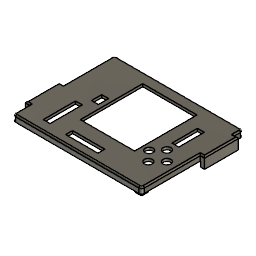
_Top Cover HiLetGo LCD.2d9b06c0-f316-4b58-bc27-3410c5de609b (Autodesk Fusion 360 design; units mm, degrees)
Autodesk Fusion 360 part; units mm, degrees
imported_body "Derived Base Feature2" makes body 1
imported_body "Derived Base Feature3" makes body 2
imported_body "Derived Base Feature4" makes body 3
imported_body "Derived Base Feature5" makes body 4
imported_body "Derived Base Feature6" makes body 5
imported_body "Derived Base Feature7" makes body 6
imported_body "Source Assembly: Context1(Enclosure)" makes body 7
sketch "Sketch1" plane through (0, 0, 38.1) normal (0, 0, 1) x (-1, 0, 0)
  line L0 (59.055, -28.1321) -> (60.325, -26.8621)
  line L1 (60.325, -26.8621) -> (60.325, -7.8121)
  line L2 (60.325, -7.8121) -> (59.055, -6.5421)
  line L3 (59.055, -6.5421) -> (59.055, 11.6667)
  arc A0 (59.055, 11.6667) -> (57.785, 12.9367) centre (57.785, 11.6667) ccw
  line L4 (57.785, 12.9367) -> (-57.785, 12.9367)
  arc A1 (-57.785, 12.9367) -> (-59.055, 11.6667) centre (-57.785, 11.6667) ccw
  line L5 (-59.055, 11.6667) -> (-59.055, -42.6733)
  line L6 (-59.055, -42.6733) -> (-60.325, -43.9433)
  line L7 (-60.325, -43.9433) -> (-60.325, -69.3433)
  line L8 (-60.325, -69.3433) -> (-59.055, -70.6133)
  line L9 (-59.055, -70.6133) -> (-59.055, -78.5033)
  arc A2 (-59.055, -78.5033) -> (-57.785, -79.7733) centre (-57.785, -78.5033) ccw
  line L10 (-57.785, -79.7733) -> (57.785, -79.7733)
  arc A3 (57.785, -79.7733) -> (59.055, -78.5033) centre (57.785, -78.5033) ccw
  line L11 (59.055, -78.5033) -> (59.055, -28.1321)
  line L12 (58.15, 12.0317) -> (58.15, -78.8683)
  line L13 (58.15, -78.8683) -> (-58.15, -78.8683)
  line L14 (-58.15, -78.8683) -> (-58.15, 12.0317)
  line L15 (-58.15, 12.0317) -> (58.15, 12.0317)
  line L16 (-57.785, -81.0433) -> (57.785, -81.0433)
  arc A4 (57.785, -81.0433) -> (60.325, -78.5033) centre (57.785, -78.5033) ccw
  line L17 (60.325, -78.5033) -> (60.325, -26.8621)
  line L18 (60.325, -7.8121) -> (60.325, 11.6667)
  arc A5 (60.325, 11.6667) -> (57.785, 14.2067) centre (57.785, 11.6667) ccw
  line L19 (57.785, 14.2067) -> (-57.785, 14.2067)
  arc A6 (-57.785, 14.2067) -> (-60.325, 11.6667) centre (-57.785, 11.6667) ccw
  line L20 (-60.325, 11.6667) -> (-60.325, -43.9433)
  line L21 (-60.325, -69.3433) -> (-60.325, -78.5033)
  arc A7 (-60.325, -78.5033) -> (-57.785, -81.0433) centre (-57.785, -78.5033) ccw
  line L22 (-60.325, -40.7683) -> (-64.2937, -40.7683)
  line L23 (-64.2937, -40.7683) -> (-64.2937, -72.5183)
  line L24 (-64.2937, -72.5183) -> (-60.325, -72.5183)
  line L25 (-60.325, -72.5183) -> (-60.325, -40.7683)
  line L26 (-62.7062, -46.3246) -> (-62.7062, -66.9621)
  line L27 (60.325, -33.2121) -> (64.2937, -33.2121)
  line L28 (64.2937, -33.2121) -> (64.2937, -1.4621)
  line L29 (64.2937, -1.4621) -> (60.325, -1.4621)
  line L30 (60.325, -1.4621) -> (60.325, -33.2121)
  line L31 (62.7063, -24.4808) -> (62.7063, -10.1933)
  line L32 (60.625, -33.2121) -> (60.625, -1.4621)
  line L33 (60.325, -78.8683) -> (60.325, 12.0317)
  line L34 (-60.625, -72.5183) -> (-60.625, -40.7683)
  line L35 (15.0813, -72.1533) -> (-21.4312, -72.1533) construction
  line L36 (-21.4312, -72.1533) -> (-21.4312, -15.0033) construction
  line L37 (-21.4312, -15.0033) -> (15.0813, -15.0033) construction
  line L38 (15.0813, -15.0033) -> (15.0813, -72.1533) construction
  line L39 (15.0813, -65.8033) -> (-21.4312, -65.8033) construction
  line L40 (-21.4312, -65.8033) -> (-21.4312, -26.1158) construction
  line L41 (-21.4312, -26.1158) -> (15.0813, -26.1158) construction
  line L42 (15.0813, -26.1158) -> (15.0813, -65.8033) construction
  line L43 (18.6531, -0.0808) -> (-11.5094, -0.0808)
  line L44 (-11.5094, -0.0808) -> (-11.5094, 6.2692)
  line L45 (-11.5094, 6.2692) -> (18.6531, 6.2692)
  line L46 (18.6531, 6.2692) -> (18.6531, -0.0808)
  line L47 (34.1312, -42.9433) -> (27.7812, -42.9433)
  line L48 (27.7812, -42.9433) -> (27.7812, -33.4183)
  line L49 (27.7812, -33.4183) -> (34.1312, -33.4183)
  line L50 (34.1312, -33.4183) -> (34.1312, -42.9433)
  line L51 (-38.1, -60.4058) -> (-44.45, -60.4058)
  line L52 (-44.45, -60.4058) -> (-44.45, -36.5933)
  line L53 (-44.45, -36.5933) -> (-38.1, -36.5933)
  line L54 (-38.1, -36.5933) -> (-38.1, -60.4058)
  circle A8 centre (-33.3375, -19.9246) radius 3.175
  circle A9 centre (-33.3375, -19.9246) radius 5.5562
  circle A10 centre (-41.275, -28.6558) radius 3.175
  circle A11 centre (-41.275, -28.6558) radius 5.5562
  circle A12 centre (-50.8, -19.1308) radius 3.175
  circle A13 centre (-50.8, -19.1308) radius 5.5562
  circle A14 centre (-42.0687, -10.3996) radius 3.175
  circle A15 centre (-42.0687, -10.3996) radius 5.5562
  circle A16 centre (-41.275, -28.6558) radius 3.675
  circle A17 centre (-33.3375, -19.9246) radius 3.675
  circle A18 centre (-50.8, -19.1308) radius 3.675
  circle A19 centre (-42.0687, -10.3996) radius 3.675
  line L55 (41.275, 4.6817) -> (34.925, 4.6817)
  line L56 (34.925, 4.6817) -> (34.925, -25.4808)
  line L57 (34.925, -25.4808) -> (41.275, -25.4808)
  line L58 (41.275, -25.4808) -> (41.275, 4.6817)
  line L59 (-21.9312, -72.6533) -> (-21.9312, -14.5033) construction
  line L60 (-21.9312, -14.5033) -> (15.5813, -14.5033) construction
  line L61 (15.5813, -14.5033) -> (15.5813, -72.6533) construction
  line L62 (15.5813, -72.6533) -> (-21.9312, -72.6533) construction
  line L63 (57.95, -78.6683) -> (51.6, -78.6683)
  line L64 (51.6, -78.6683) -> (51.6, -76.1283)
  line L65 (51.6, -76.1283) -> (55.41, -76.1283)
  line L66 (57.95, -78.6683) -> (57.95, -72.3183)
  line L67 (57.95, -72.3183) -> (55.41, -72.3183)
  line L68 (55.41, -72.3183) -> (55.41, -76.1283)
  line L69 (51.6, -78.6683) -> (51.6, -78.8683)
  line L70 (57.95, -72.3183) -> (58.15, -72.3183)
  line L71 (85.0596, -33.4183) -> (-85.0118, -33.4183) construction
  line L72 (51.6, 11.8317) -> (51.6, 12.0317)
  line L73 (57.95, 11.8317) -> (51.6, 11.8317)
  line L74 (57.95, 5.4817) -> (55.41, 5.4817)
  line L75 (55.41, 5.4817) -> (55.41, 9.2917)
  line L76 (57.95, 11.8317) -> (57.95, 5.4817)
  line L77 (57.95, 5.4817) -> (58.15, 5.4817)
  line L78 (51.6, 9.2917) -> (55.41, 9.2917)
  line L79 (51.6, 11.8317) -> (51.6, 9.2917)
  line L80 (0, -87.3252) -> (0, 24.4348) construction
  line L81 (-57.95, 5.4817) -> (-58.15, 5.4817)
  line L82 (-57.95, 5.4817) -> (-55.41, 5.4817)
  line L83 (-57.95, 11.8317) -> (-57.95, 5.4817)
  line L84 (-55.41, 5.4817) -> (-55.41, 9.2917)
  line L85 (-51.6, 9.2917) -> (-55.41, 9.2917)
  line L86 (-51.6, 11.8317) -> (-51.6, 9.2917)
  line L87 (-57.95, 11.8317) -> (-51.6, 11.8317)
  line L88 (-51.6, 11.8317) -> (-51.6, 12.0317)
  line L89 (23.8363, -71.0658) -> (-26.9637, -71.0658)
  line L90 (-26.9637, -71.0658) -> (-26.9637, -12.6458)
  line L91 (-26.9637, -12.6458) -> (23.8363, -12.6458)
  line L92 (23.8363, -12.6458) -> (23.8363, -71.0658)
  point P0 (-64.2937, -56.6433)
  point P1 (-62.7062, -56.6433)
  point P2 (64.2937, -17.3371)
  point P3 (62.7063, -17.3371)
  point P4 (58.15, -33.4183)
  point P5 (-58.15, -33.4183)
  point P6 (0, -78.8683)
  dimension "d3" = 31.75
  dimension "d4" = 3.9688
  dimension "d5" = 31.75
  dimension "d6" = 3.9688
  dimension "d9" = 0.3
  dimension "d10" = 0.3
  dimension "d23" = 57.15
  dimension "d24" = 36.5125
  dimension "d25" = 29.21
  dimension "d26" = 38.8938
  dimension "d27" = 39.6875
  dimension "d28" = 11.1125
  dimension "d29" = 6.35
  dimension "d30" = 7.9375
  dimension "d31" = 41.6719
  dimension "d32" = 30.1625
  dimension "d33" = 9.525
  dimension "d34" = 6.35
  dimension "d35" = 47.625
  dimension "d36" = 26.1938
  dimension "d37" = 6.35
  dimension "d38" = 15.875
  dimension "d39" = 23.8125
  dimension "d40" = 50.8
  dimension "d41" = 0.5
  dimension "d42" = 0.5
  dimension "d43" = 0.5
  dimension "d44" = 0.5
  dimension "d45" = 6.35
  dimension "d46" = 30.1625
  dimension "d47" = 19.05
  dimension "d48" = 9.525
  dimension "d50" = -0.5
  dimension "d54" = 6.35
  dimension "d55" = 3.81
  dimension "d56" = 6.35
  dimension "d57" = 2.54
  dimension "d58" = 3.81
  dimension "d59" = 0.2
  dimension "d60" = 0.2
  dimension "d65" = 50.8
  dimension "d66" = 58.42
  dimension "d67" = 1.5875
  dimension "d68" = 8.255
  constraint horizontal L22
  constraint vertical L23
  constraint horizontal L24
  constraint vertical L25
  constraint coincident L20 L22.start
  constraint midpoint L23 P0
  constraint midpoint L26 P1
  constraint horizontal P0 P1
  constraint horizontal L27
  constraint vertical L28
  constraint horizontal L29
  constraint vertical L30
  constraint coincident L17 L27.start
  constraint midpoint L28 P2
  constraint midpoint L31 P3
  constraint horizontal P2 P3
  constraint coincident L27 L32.start
  constraint coincident L29 L32.end
  constraint perpendicular L29 L32
  constraint coincident L24 L34.start
  constraint coincident L22 L34.end
  constraint perpendicular L22 L34
  constraint horizontal L35
  constraint vertical L36
  constraint horizontal L37
  constraint vertical L38
  constraint horizontal L39
  constraint vertical L40
  constraint horizontal L41
  constraint vertical L42
  constraint coincident L36 L40.end
  constraint coincident L38 L39.start
  constraint horizontal L43
  constraint vertical L44
  constraint horizontal L45
  constraint vertical L46
  constraint horizontal L47
  constraint vertical L48
  constraint horizontal L49
  constraint vertical L50
  constraint horizontal L51
  constraint vertical L52
  constraint horizontal L53
  constraint vertical L54
  constraint horizontal L55
  constraint vertical L56
  constraint horizontal L57
  constraint vertical L58
  constraint horizontal L63
  constraint perpendicular L63 L64
  constraint perpendicular L64 L65
  constraint perpendicular L63 L66
  constraint perpendicular L66 L67
  constraint coincident L13 L69.end
  constraint perpendicular L13 L69
  constraint coincident L12 L70.end
  constraint perpendicular L12 L70
  constraint midpoint L12 P4
  constraint coincident L71 P4
  constraint midpoint L14 P5
  constraint coincident L71 P5
  constraint symmetric L63.start L71 L73.start
  constraint symmetric L63.end L71 L72.start
  constraint symmetric L64.end L71 L78.start
  constraint symmetric L65.end L71 L75.end
  constraint symmetric L66.end L71 L74.start
  constraint symmetric L67.end L71 L74.end
  constraint symmetric L69.end L71 L72.end
  constraint symmetric L70.end L71 L77.end
  constraint perpendicular L43 L80
  constraint midpoint L13 P6
  constraint coincident L80 P6
  constraint symmetric L72.start L80 L86.start
  constraint symmetric L72.end L80 L88.end
  constraint symmetric L73.start L80 L83.start
  constraint symmetric L74.start L80 L81.start
  constraint symmetric L74.end L80 L82.end
  constraint symmetric L75.end L80 L84.end
  constraint symmetric L77.end L80 L81.end
  constraint symmetric L78.start L80 L85.start
  constraint horizontal L89
  constraint vertical L90
  constraint horizontal L91
  constraint vertical L92
  measures "d3" distance of L22.end L23.end
  measures "d4" distance of L23.end L24.end
  measures "d5" distance of L27.end L28.end
  measures "d6" distance of L27.start L27.end
  measures "d9" distance of L32 L33
  measures "d10" distance of L25 L34
  measures "d23" distance of L35.start L37.end
  measures "d24" distance of L35.start L35.end
  measures "d25" distance of L19 L37
  measures "d26" distance of L20 L36
  measures "d27" distance of L39 L41
  measures "d28" distance of L37 L41
  measures "d29" distance of L43.start L45.end
  measures "d30" distance of L19 L45
  measures "d31" distance of L18 L46
  measures "d32" distance of L43.start L43.end
  measures "d33" distance of L47.end L48.end
  measures "d34" distance of L48.end L49.end
  measures "d35" distance of L19 L49
  measures "d36" distance of L33 L50
  measures "d37" distance of L52.end L53.end
  measures "d38" distance of L20 L52
  measures "d39" distance of L51.end L52.end
  measures "d40" distance of L19 L53
  measures "d45" distance of L55.start L55.end
  measures "d46" distance of L55.end L56.end
  measures "d47" distance of L33 L58
  measures "d48" distance of L19 L55
  measures "d54" distance of L63.start L63.end
  measures "d55" distance of L64.end L65.end
  measures "d56" distance of L63.start L66.end
  measures "d57" distance of L66.end L67.end
  measures "d58" distance of L65.end L67.end
  measures "d59" distance of L13 L63
  measures "d60" distance of L12 L66
  measures "d65" distance of L89.start L89.end
  measures "d66" distance of L89.start L91.end
  measures "d67" distance of L62 L89
  measures "d68" distance of L61 L92
extrude "Extrude5" add sketch "Sketch1" along normal blind 3.175 separate body contours L0 L1 L2 L3 A0 L4 A1 L5 L6 L7 L8 L9 A2 L10 A3 L11 L25 L30 L33 | L0 L8 L9 A2 L10 A3 L11 L16 A4 L17 L21 A7 L25 L30 L33 | L1 L17 L18 L27 L29 L30 L32 L33 | L2 L3 A0 L4 A1 L5 L6 L18 A5 L19 A6 L20 L25 L30 L33 | L27 L28 L29 L32 | L7 L20 L21 L22 L24 L25 L34 | L22 L23 L24 L34 | L12 L15 L72 L73 L76 L77 | L12 L13 L63 L66 L69 L70 | L73 L74 L75 L76 L78 L79 | L14 L15 L81 L83 L87 L88 | L63 L64 L65 L66 L67 L68 | L82 L83 L84 L85 L86 L87 makes body 8
extrude "Extrude1" add sketch "Sketch1" along normal blind 2.54 from surface at 3.175 contours L0 L1 L2 L3 A0 L4 A1 L5 L6 L7 L8 L9 A2 L10 A3 L11 L25 L30 L33 | L0 L8 L9 A2 L10 A3 L11 L16 A4 L17 L21 A7 L25 L30 L33 | L1 L17 L18 L27 L29 L30 L32 L33 | L2 L3 A0 L4 A1 L5 L6 L18 A5 L19 A6 L20 L25 L30 L33 | L27 L28 L29 L32 | L7 L20 L21 L22 L24 L25 L34 | L22 L23 L24 L34 | L12 L15 L72 L73 L76 L77 | L12 L13 L14 L15 L64 L65 L67 L68 L69 L70 L72 L74 L75 L77 L78 L79 L81 L82 L84 L85 L86 L88 | L12 L13 L63 L66 L69 L70 | L73 L74 L75 L76 L78 L79 | L14 L15 L81 L83 L87 L88 | L63 L64 L65 L66 L67 L68 | L82 L83 L84 L85 L86 L87 | A9 | A11 | A13 | A15 bodies 8
extrude "Extrude2" add sketch "Sketch1" against normal blind 4.7625 separate body contours L27 L28 L29 L32 | L22 L23 L24 L34 makes body 9 at (-60.625, 22.6287, 34.925) makes body 10 at (64.2937, 51.3517, 34.925)
sketch "sketch 1168" plane through (-60.325, 0, 6.35) normal (1, 0, 0) x (0, 1, 0)
  line L0 (20.312, 0) -> (20.312, -3.175)
  line L1 (20.312, -3.175) -> (78.8683, -3.175)
  line L2 (78.8683, -3.175) -> (78.8683, 31.75)
  line L3 (78.8683, 31.75) -> (-12.0317, 31.75)
  line L4 (-12.0317, 31.75) -> (-12.0317, 20.468)
  spline S0 degree 3 poles (5.7434, 20.4049) (4.1602, 20.592) (2.431, 20.6756) (-3.2122, 20.8085) (-8.0065, 20.625) (-12.0317, 20.468) knots -1.695803 -1.695803 -1.695803 -1.695803 -1.238024 -1.238024 -0.049614 -0.049614 -0.049614 -0.049614
  spline S1 degree 3 poles (20.2542, 16.6769) (18.4736, 17.4882) (15.9586, 18.1286) (9.6823, 19.709) (7.9499, 20.1441) (5.7434, 20.4049) knots -2.351658 -2.351658 -2.351658 -2.351658 -0.666575 -0.666575 0 0 0 0
  spline S2 degree 3 poles (23.9917, 13.1288) (23.7587, 13.6736) (23.4127, 14.3018) (22.095, 15.6928) (21.2089, 16.242) (20.2542, 16.6769) knots -0.574521 -0.574521 -0.574521 -0.574521 -0.314729 -0.314729 0 0 0 0
  spline S3 degree 3 poles (24.9586, 10.1587) (24.5607, 11.3167) (24.3713, 12.2408) (23.9917, 13.1288) knots -0.289722 -0.289722 -0.289722 -0.289722 0 0 0 0
  spline S4 degree 3 poles (24.6891, 10.1614) (24.7346, 10.161) (24.78, 10.1606) (24.8699, 10.1597) (24.9143, 10.1592) (24.9586, 10.1587) knots -0.02718 -0.02718 -0.02718 -0.02718 -0.013541 -0.013541 -0.000226 -0.000226 -0.000226 -0.000226
  line L5 (24.6102, 9.9104) -> (24.6891, 10.1614)
  spline S5 degree 3 poles (25.015, 9.9064) (24.9481, 9.9072) (24.8811, 9.9079) (24.7462, 9.9092) (24.6782, 9.9098) (24.6102, 9.9104) knots -0.040486 -0.040486 -0.040486 -0.040486 -0.020398 -0.020398 0 0 0 0
  spline S6 degree 3 poles (20.312, 0) (20.985, 0.4196) (21.6323, 0.8894) (22.7162, 1.8686) (23.1736, 2.3651) (24.2324, 3.8634) (24.5842, 4.8027) (25.2036, 7.3749) (25.1188, 8.8356) (25.015, 9.9064) knots -0.713353 -0.713353 -0.713353 -0.713353 -0.595622 -0.595622 -0.495533 -0.495533 -0.323538 -0.323538 -0.002781 -0.002781 -0.002781 -0.002781
  line L6 (7.8121, 31.75) -> (26.8621, 31.75)
  line L7 (26.8621, 31.75) -> (26.8621, 26.9875)
  line L8 (26.8621, 26.9875) -> (7.8121, 26.9875)
  line L9 (7.8121, 26.9875) -> (7.8121, 31.75)
  line L10 (14.3249, -6.35) -> (14.3249, 0)
  spline S7 degree 3 poles (18.9957, 9.5628) (19.1452, 8.8795) (19.2886, 8.2267) (19.3768, 6.9383) (19.3535, 6.1927) (18.894, 4.6274) (18.5281, 3.8259) (17.1565, 2.1284) (16.1672, 1.2251) (14.3249, 0) knots -3.705715 -3.705715 -3.705715 -3.705715 -2.605275 -2.605275 -1.649976 -1.649976 -0.868848 -0.868848 -0.117348 -0.117348 -0.117348 -0.117348
  line L11 (18.5587, 9.5512) -> (18.9957, 9.5628)
  line L12 (18.6412, 9.8055) -> (18.5587, 9.5512)
  line L13 (18.9245, 9.8131) -> (18.6412, 9.8055)
  spline S8 degree 3 poles (11.9392, 16.9539) (13.2511, 16.4171) (14.3702, 15.8494) (16.109, 14.6196) (16.735, 14.0136) (18.0844, 12.2103) (18.4999, 11.0258) (18.9245, 9.8131) knots -0.898912 -0.898912 -0.898912 -0.898912 -0.624615 -0.624615 -0.390602 -0.390602 -0.004883 -0.004883 -0.004883 -0.004883
  spline S9 degree 3 poles (4.6437, 19.17) (6.2001, 18.8891) (7.9332, 18.4318) (10.8472, 17.3822) (11.4058, 17.1722) (11.9392, 16.9539) knots -0.934389 -0.934389 -0.934389 -0.934389 -0.172902 -0.172902 0 0 0 0
  spline S10 degree 3 poles (-14.2067, 19.4952) (-7.065, 19.7734) (-4.9162, 19.7975) (0.2422, 19.707) (2.5779, 19.5427) (4.6437, 19.17) knots -1.21446 -1.21446 -1.21446 -1.21446 -0.629755 -0.629755 0 0 0 0
  line L14 (-14.2067, 19.4952) -> (-14.2067, 31.75)
  line L15 (-14.2067, 31.75) -> (81.0433, 31.75)
  line L16 (81.0433, 31.75) -> (81.0433, -6.35)
  line L17 (81.0433, -6.35) -> (14.3249, -6.35)
extrude "Extrude3" cut sketch "sketch 1168" against normal blind 4.7625 draft -45 from surface at -0.3 contours L3 L6 L7 L8 L9 L15 bodies 9
sketch "sketch 1759" plane through (60.325, 0, 6.35) normal (-1, 0, 0) x (0, -1, 0)
  line L0 (-20.3121, -3.175) -> (-20.3121, 0)
  spline S0 degree 3 poles (-25.0151, 9.9065) (-25.0979, 9.0511) (-25.2498, 7.0718) (-24.3902, 4.3138) (-24.0256, 3.5358) (-22.7188, 1.7749) (-21.6836, 0.8552) (-20.3121, 0) knots -1.87536 -1.87536 -1.87536 -1.87536 -0.911021 -0.911021 -0.526686 -0.526686 -0.031937 -0.031937 -0.031937 -0.031937
  spline S1 degree 3 poles (-24.6102, 9.9104) (-24.6791, 9.9099) (-24.7479, 9.9092) (-24.8828, 9.9079) (-24.949, 9.9072) (-25.0151, 9.9065) knots -0.040991 -0.040991 -0.040991 -0.040991 -0.020342 -0.020342 -0.000506 -0.000506 -0.000506 -0.000506
  line L1 (-24.6892, 10.1614) -> (-24.6102, 9.9104)
  spline S2 degree 3 poles (-24.9587, 10.1588) (-24.9141, 10.1592) (-24.8694, 10.1597) (-24.7796, 10.1606) (-24.7344, 10.161) (-24.6892, 10.1614) knots -0.026954 -0.026954 -0.026954 -0.026954 -0.013566 -0.013566 0 0 0 0
  spline S3 degree 3 poles (-23.9487, 13.0533) (-24.3822, 12.1904) (-24.5675, 11.2969) (-24.9587, 10.1588) knots -0.362462 -0.362462 -0.362462 -0.362462 -0.000942 -0.000942 -0.000942 -0.000942
  spline S4 degree 3 poles (-19.3919, 16.7881) (-20.5523, 16.2621) (-21.6214, 15.6478) (-23.2385, 14.2444) (-23.6656, 13.6166) (-23.9487, 13.0533) knots -0.398015 -0.398015 -0.398015 -0.398015 -0.189134 -0.189134 0 0 0 0
  spline S5 degree 3 poles (12.0317, 20.7153) (11.9537, 20.7168) (11.8757, 20.7183) (11.5581, 20.7246) (11.3187, 20.7294) (10.61, 20.7438) (10.1392, 20.7537) (8.7283, 20.7839) (7.7449, 20.8059) (5.6849, 20.8535) (5.3766, 20.8616) (2.4879, 20.9241) (0.349, 20.9452) (-3.1682, 20.7741) (-4.8643, 20.6391) (-8.3884, 20.0368) (-9.8842, 19.7165) (-13.8921, 18.7442) (-17.0403, 17.854) (-19.3919, 16.7881) knots -4.093208 -4.093208 -4.093208 -4.093208 -4.069141 -4.069141 -3.995237 -3.995237 -3.850451 -3.850451 -3.559151 -3.559151 -3.211336 -3.211336 -2.015115 -2.015115 -1.239815 -1.239815 -0.774566 -0.774566 0 0 0 0
  line L2 (12.0317, 20.7153) -> (12.0317, 31.75)
  line L3 (12.0317, 31.75) -> (-78.8683, 31.75)
  line L4 (-78.8683, 31.75) -> (-78.8683, -3.175)
  line L5 (-78.8683, -3.175) -> (-20.3121, -3.175)
  line L6 (-69.3433, 31.75) -> (-43.9433, 31.75)
  line L7 (-43.9433, 31.75) -> (-43.9433, 26.9875)
  line L8 (-43.9433, 26.9875) -> (-69.3433, 26.9875)
  line L9 (-69.3433, 26.9875) -> (-69.3433, 31.75)
  line L10 (-14.3267, 0) -> (-14.3267, -6.35)
  line L11 (-14.3267, -6.35) -> (-81.0433, -6.35)
  line L12 (-81.0433, -6.35) -> (-81.0433, 31.75)
  line L13 (-81.0433, 31.75) -> (14.2067, 31.75)
  line L14 (14.2067, 31.75) -> (14.2067, 19.7415)
  spline S6 degree 3 poles (-11.809, 17.0428) (-10.6277, 17.5559) (-9.4045, 17.9855) (-7.2632, 18.6871) (-6.0003, 19.0317) (-2.9908, 19.6356) (-1.3381, 19.8178) (2.8213, 19.9698) (4.9046, 19.9247) (10.0799, 19.8211) (11.207, 19.7987) (13.2957, 19.7586) (13.7074, 19.7516) (14.2067, 19.7415) knots -3.119715 -3.119715 -3.119715 -3.119715 -2.692781 -2.692781 -2.045016 -2.045016 -1.216358 -1.216358 -0.396749 -0.396749 -0.245718 -0.245718 -0.057039 -0.057039 -0.057039 -0.057039
  spline S7 degree 3 poles (-18.9349, 9.8153) (-18.6903, 10.511) (-18.4431, 11.2059) (-17.7565, 12.563) (-17.3022, 13.2686) (-15.6846, 14.9295) (-14.2751, 15.9716) (-11.809, 17.0428) knots -2.051239 -2.051239 -2.051239 -2.051239 -1.419817 -1.419817 -0.806611 -0.806611 0 0 0 0
  line L15 (-18.6534, 9.8082) -> (-18.9349, 9.8153)
  line L16 (-18.5715, 9.5539) -> (-18.6534, 9.8082)
  line L17 (-19.0058, 9.565) -> (-18.5715, 9.5539)
  spline S8 degree 3 poles (-14.3267, 0) (-15.4198, 0.7273) (-16.1601, 1.3022) (-17.306, 2.3262) (-17.9829, 3.0358) (-19.0011, 4.7957) (-19.2149, 5.6048) (-19.4608, 7.4616) (-19.2368, 8.4947) (-19.0058, 9.565) knots -0.871235 -0.871235 -0.871235 -0.871235 -0.701314 -0.701314 -0.51379 -0.51379 -0.330092 -0.330092 -0.00152 -0.00152 -0.00152 -0.00152
extrude "Extrude4" cut sketch "sketch 1759" against normal blind 4.7625 draft -45 from surface at -0.3 contours L3 L6 L7 L8 L9 L13 bodies 10
sketch "Sketch2" plane through (-60.325, 0, 0) normal (-1, 0, 0) x (0, -1, 0)
  line L0 (-78.5033, 38.1) -> (-33.2121, 38.1)
  line L1 (-33.2121, 38.1) -> (-33.2121, 43.815)
  line L2 (-33.2121, 43.815) -> (-78.5033, 43.815)
  line L3 (-78.5033, 43.815) -> (-78.5033, 38.1)
  line L4 (-71.0406, 29.5963) -> (-71.0406, 35.9463)
  line L5 (-71.0406, 35.9463) -> (-56.896, 35.9463)
  line L6 (-56.896, 29.5963) -> (-71.0406, 29.5963)
  line L7 (-56.896, 35.9463) -> (-56.896, 29.5963)
  line L8 (-71.0406, 38.1) -> (-56.896, 38.1)
  line L9 (-56.896, 38.1) -> (-56.896, 42.0688)
  line L10 (-56.896, 42.0688) -> (-71.0406, 42.0688)
  line L11 (-71.0406, 42.0688) -> (-71.0406, 38.1)
  dimension "d20" = 3.9688
  constraint horizontal L8
  constraint vertical L9
  constraint horizontal L10
  constraint vertical L11
  constraint coincident L0 L8.start
  constraint collinear L4 L11
  constraint collinear L7 L9
  measures "d20" distance of L8.end L9.end
extrude "Extrude6" cut sketch "Sketch2" against normal blind 3.175 contours L0 L8 L9 L10 L11 bodies 8
ref_plane "WorkPlane1" through (1.9942, 38.3352, 47.5475) normal (0, 0, 1) x (1, 0, 0)
fillet "Fillet1" radius 1.27 16 edges at (-60.325, -5.1023, 43.815) (-59.5811, -13.4627, 43.815) (0, -14.2067, 43.815) (59.5811, -13.4627, 43.815) (60.325, 14.5508, 43.815) (-62.3094, 1.4621, 43.815) (-64.2937, 17.3371, 43.815) (-62.3094, 33.2121, 43.815) (60.325, 75.5108, 43.815) (59.5811, 80.2994, 43.815) (0, 81.0433, 43.815) (-59.5811, 80.2994, 43.815) (-60.325, 55.8577, 43.815) (62.3094, 72.5183, 43.815) (64.2937, 56.6433, 43.815) (62.3094, 40.7683, 43.815) on bodies 8
combine "Combine1" operation add target body 8 tool bodies 10 9
extrude "Extrude7" add sketch "Sketch1" against normal blind 3.175 contours L63 L64 L65 L66 L67 L68 | L82 L83 L84 L85 L86 L87 bodies 8
fillet "Fillet2" radius 1.27 5 edges at (55.41, -9.2917, 38.1) (57.95, -11.8317, 36.5125) (-57.95, 78.6683, 36.5125) (-55.41, 76.1283, 38.1) (-55.41, -9.2917, 39.6875) on bodies 8
hidden bodies 7 1 2 3 4 5 6
equation "d4 = ( 5 / 32 ) * 1 in"
equation "d6 = ( 5 / 32 ) * 1 in"
equation "d7 = ( -3 / 16 ) * 1 in"
equation "d12 = ( -3 / 16 ) * 1 in"
equation "d15 = ( -3 / 16 ) * 1 in"
equation "d20 = ( 5 / 32 ) * 1 in"
equation "d24 = 1 in + ( 7 / 16 ) * 1 in"
equation "d26 = 1 in + ( 17 / 32 ) * 1 in"
equation "d27 = 1 in + ( 9 / 16 ) * 1 in"
equation "d28 = ( 7 / 16 ) * 1 in"
equation "d30 = ( 5 / 16 ) * 1 in"
equation "d31 = 1 in + ( 5 / 8 ) * 1 in + ( 1 / 64 ) * 1 in"
equation "d32 = ( 2 in + ( 13 / 16 ) * 1 in ) - ( 1 in + ( 5 / 8 ) * 1 in )"
equation "d34 = ( 1 / 4 ) * 1 in"
equation "d35 = 1 in + ( 7 / 8 ) * 1 in"
equation "d36 = 1 in + ( 1 / 32 ) * 1 in"
equation "d37 = ( 1 / 4 ) * 1 in"
equation "d38 = ( 5 / 8 ) * 1 in"
equation "d39 = ( 15 / 16 ) * 1 in"
equation "d45 = ( 1 / 4 ) * 1 in"
equation "d46 = 1.25 in - ( 1 / 16 ) * 1 in"
equation "d47 = ( 3 / 4 ) * 1 in"
equation "d48 = ( 3 / 8 ) * 1 in"
equation "d49 = ( 11 / 16 ) * 1 in"
equation "d67 = ( 1 / 16 ) * 1 in"
named bodies: "Body51", "Body51 (Context1)", "Body51 (1)", "Body51 (Context2)", "Body1 (Context2)", "Body1 (1) (Context2)", "Body1 (2) (Context2)", "Body1 (3) (Context2)", "ECE319-Lab9-PCB-model (44)", "ECE319-Lab9-PCB-model (44) (Context2)"
